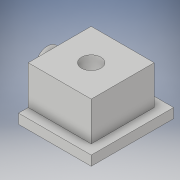
# Autodesk Inventor part: WackyPlug1.75
Saved by Autodesk Inventor 2018.3 (Build 223284000, 284)
## iProperties
Created: 2020-01-21
Part Number: WackyPlug1.75
Material: Generic
Document SubType Name: Modeling
Designer: 22perngrac
Density: 1 g/cm^3
Appearance: Default
Mass: 57.4742 g
Surface Area: 120.738 cm^2
Volume: 57.4742 cm^3
Author: 22perngrac
Autodesk Inventor part; units mm, degrees
ref_plane "YZ Plane" through (0, 0, 0) normal (1, 0, 0) x (0, 1, 0)
ref_plane "XZ Plane" through (0, 0, 0) normal (0, 1, 0) x (-1, 0, 0)
ref_plane "XY Plane" through (0, 0, 0) normal (0, 0, 1) x (1, 0, 0)
sketch "Sketch1" plane through (0, 0, 0) normal (0, 1, 0) x (-1, 0, 0)
  line L0 (0, 0) -> (42.8625, 0)
  line L1 (42.8625, 0) -> (42.8625, -44.45)
  line L2 (42.8625, -44.45) -> (0, -44.45)
  line L3 (0, -44.45) -> (0, 0)
  dimension "d0" = 44.45
  dimension "d1" = 42.8625
  constraints: 8 end point, 2 parallel, 1 horizontal, 1 perpendicular
  measures "d0" distance of L0.end L1.end
  measures "d1" distance of L1.end L2.end
extrude "Extrusion1" add sketch "Sketch1" along normal blind 31.75
sketch "Sketch2" plane through (-42.8625, 0, 0) normal (0, 0, 1) x (1, 0, 0)
  line L0 (0, 0) -> (0, 31.75) projected
  line L1 (42.8625, 0) -> (42.8625, 31.75) projected
  line L2 (42.8625, 0) -> (0, 0) projected
  line L3 (0, 6.35) -> (42.8625, 6.35)
  line L4 (42.8625, 6.35) -> (42.8625, 31.75)
  line L5 (42.8625, 31.75) -> (0, 31.75)
  line L6 (0, 31.75) -> (0, 6.35)
  dimension "d5" = 6.35
  constraints: 8 end point, 2 parallel, 1 horizontal, 1 perpendicular, 1 point on line
  measures "d5" distance between parallel lines of L2 L3
extrude "Extrusion2" cut sketch "Sketch2" against normal blind 1.5875 contours L0 L5 L1 L3
sketch "Sketch3" plane through (0, 0, 0) normal (1, 0, 0) x (0, 0, -1)
  line L0 (1.5875, 31.75) -> (1.5875, 6.35) projected
  line L1 (44.45, 0) -> (44.45, 31.75) projected
  line L2 (1.5875, 6.35) -> (44.45, 6.35)
  line L3 (44.45, 6.35) -> (44.45, 31.75)
  line L4 (44.45, 31.75) -> (1.5875, 31.75)
  line L5 (1.5875, 31.75) -> (1.5875, 6.35)
  point P0 (0, 0)
  constraints: 8 end point, 2 parallel, 1 horizontal, 1 perpendicular
extrude "Extrusion3" cut sketch "Sketch3" against normal blind 1.5875
sketch "Sketch9" plane through (0, 31.75, 0) normal (0, 1, 0) x (1, 0, 0)
  line L0 (0, 44.45) -> (0, 0) projected
  line L1 (-1.5875, 44.45) -> (0, 44.45) projected
  point P0 (-22.225, 22.225)
  point P1 (-42.8625, 44.45)
  dimension "d23" = 22.225
  dimension "d24" = 22.225
  measures "d23" distance from line of L0 point (-22.225, 22.225)
  measures "d24" distance from line of L1 point (-22.225, 22.225)
hole "Hole1" at (-22.225, 31.75, -22.225) direction (0, -1, 0) diameter 12.7 end through all
sketch "Sketch19" plane through (0, 0, -44.45) normal (0, 0, -1) x (-1, 0, 0)
  line L0 (1.5875, 31.75) -> (42.8625, 31.75) projected
  line L1 (1.5875, 6.35) -> (42.8625, 6.35) projected
  line L2 (1.5875, 31.75) -> (42.8625, 31.75)
  line L3 (42.8625, 31.75) -> (42.8625, 6.35)
  line L4 (42.8625, 6.35) -> (1.5875, 6.35)
  line L5 (1.5875, 6.35) -> (1.5875, 31.75)
  point P0 (0, 0)
  constraints: 8 end point, 2 parallel, 1 horizontal, 1 perpendicular
extrude "Extrusion14" cut sketch "Sketch19" against normal blind 1.5875
sketch "Sketch20" plane through (-42.8625, 0, -44.45) normal (-1, 0, 0) x (0, 0, 1)
  circle A0 centre (22.225, 19.05) radius 7.9375
  line L0 (44.45, 0) -> (0, 0) projected
  line L1 (44.45, 0) -> (44.45, 6.35) projected
  dimension "d59" = 15.875
  dimension "d60" = 19.05
  dimension "d61" = 22.225
  constraints: 1 centre point
  measures "d59" diameter of A0
  measures "d60" distance from line of L0 A0.centre
  measures "d61" distance from line of A0.centre L1
extrude "Extrusion15" add sketch "Sketch20" along normal blind 7.9375
sketch "Sketch21" plane through (0, 0, -44.45) normal (0, 0, -1) x (-1, 0, 0)
  line L0 (42.8625, 6.35) -> (0, 6.35) projected
  line L1 (0, 0) -> (0, 6.35) projected
  line L2 (42.8625, 0) -> (0, 0) projected
  line L3 (42.8625, 0) -> (42.8625, 6.35) projected
  point P0 (0, 0)
extrude "Extrusion16" add sketch "Sketch21" along normal blind 4.7625
sketch "Sketch22" plane through (-42.8625, 0, 0) normal (0, 0, 1) x (1, 0, 0)
  line L0 (42.8625, 6.35) -> (0, 6.35) projected
  line L1 (0, 0) -> (0, 6.35) projected
  line L2 (42.8625, 0) -> (0, 0) projected
  line L3 (42.8625, 0) -> (42.8625, 6.35) projected
extrude "Extrusion17" add sketch "Sketch22" along normal blind 4.7625
sketch "Sketch23" plane through (0, 0, -49.2125) normal (1, 0, 0) x (0, 0, -1)
  line L0 (0, 6.35) -> (-53.975, 6.35) projected
  line L1 (-53.975, 0) -> (-53.975, 6.35) projected
  line L2 (0, 0) -> (-53.975, 0) projected
  line L3 (0, 6.35) -> (0, 0) projected
  point P0 (-49.2125, 0)
extrude "Extrusion18" add sketch "Sketch23" along normal blind 4.7625
equation "\"d24\" = d23"
body "Solid1"
